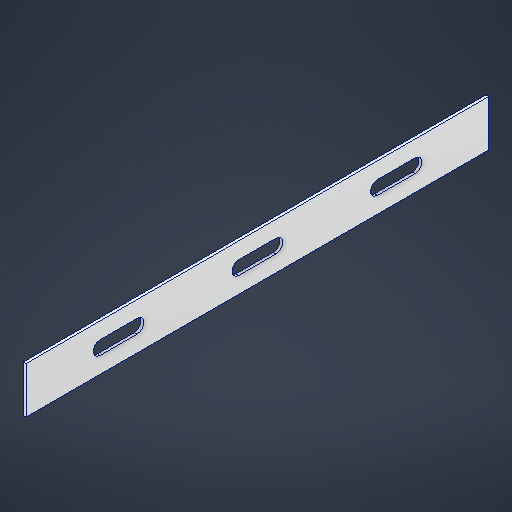
# Autodesk Inventor part: FLoor Frame, Small
Saved by Autodesk Inventor 2026 (Build 300175000, 175)
## iProperties
Created: 2025-10-29
Part Number: FLoor Frame, Small
Material: Aluminum 6061
Document SubType Name: Sheet Metal
Designer: Brandon Portillo
Density: 2.7 g/cm^3
Sheet Metal Rule: Default
Appearance: Aluminum - Flat
Author: Brandon Portillo
Autodesk Inventor part; units mm, degrees
ref_plane "YZ Plane" through (0, 0, 0) normal (1, 0, 0) x (0, 1, 0)
ref_plane "XZ Plane" through (0, 0, 0) normal (0, 1, 0) x (-1, 0, 0)
ref_plane "XY Plane" through (0, 0, 0) normal (0, 0, 1) x (1, 0, 0)
sketch "Sketch1" plane through (0, 0, 0) normal (1, 0, 0) x (0, 1, 0)
  line L0 (0, 0) -> (50, 0)
  line L1 (50, 0) -> (50, -500)
  line L2 (50, -500) -> (0, -500)
  line L3 (0, -500) -> (0, 0)
  dimension "d0" = 50
  dimension "d1" = 500
  measures "d0" distance of L1.end L2.end
  measures "d1" distance of L0.end L1.end
extrude "Plate1" add sketch "Sketch1" along normal blind 3
sketch "Sketch2" plane through (3, 0, 0) normal (1, 0, 0) x (0, 0, -1)
  line L0 (0, 50) -> (0, 0) projected
  line L1 (0, 25) -> (100, 25)
  line L2 (500, 0) -> (500, 50) projected
  line L3 (500, 25) -> (400, 25)
  line L4 (100, 25) -> (400, 25)
  line L5 (80.0463, 25) -> (119.9537, 25) construction
  line L6 (80.0463, 17.6266) -> (119.9537, 17.6266)
  line L7 (119.9537, 32.3734) -> (80.0463, 32.3734)
  arc A0 (80.0463, 32.3734) -> (80.0463, 17.6266) centre (80.0463, 25) ccw
  arc A1 (119.9537, 17.6266) -> (119.9537, 32.3734) centre (119.9537, 25) ccw
  line L8 (270.0297, 25) -> (229.9703, 25) construction
  line L9 (270.0297, 17.6266) -> (229.9703, 17.6266)
  line L10 (229.9703, 32.3734) -> (270.0297, 32.3734)
  arc A2 (270.0297, 17.6266) -> (270.0297, 32.3734) centre (270.0297, 25) ccw
  arc A3 (229.9703, 32.3734) -> (229.9703, 17.6266) centre (229.9703, 25) ccw
  line L11 (420.3445, 25) -> (379.6555, 25) construction
  line L12 (420.3445, 17.6266) -> (379.6555, 17.6266)
  line L13 (379.6555, 32.3734) -> (420.3445, 32.3734)
  arc A4 (420.3445, 17.6266) -> (420.3445, 32.3734) centre (420.3445, 25) ccw
  arc A5 (379.6555, 32.3734) -> (379.6555, 17.6266) centre (379.6555, 25) ccw
  point P0 (250, 25)
  dimension "d3" = 100
  dimension "d4" = 100
  constraints: 30 end point, 12 point on circle, 12 tangent, 6 centre point, 6 midpoint, 3 parallel, 3 point on line, 2 coincident, 2 horizontal, 1 collinear
  measures "d3" distance of L1.start L1.end
  measures "d4" distance of L3.start L3.end
extrude "Cut1" cut sketch "Sketch2" against normal blind 3
equation "\"d5\" = Thickness"
equation "\"d2\" = Thickness"
equation "\"BendRadius\" = Thickness"
equation "\"BendReliefWidth\" = Thickness"
equation "\"BendReliefDepth\" = 0.5 * Thickness"
equation "\"CornerReliefSize\" = 4 * Thickness"
equation "\"MinimumRemnant\" = 2 * Thickness"
equation "\"TransitionRadius\" = BendRadius"
equation "\"JacobiRadiusSize\" = BendRadius"
equation "\"GapSize\" = Thickness"
equation "\"Thickness\" = 3"
body "Solid1"
